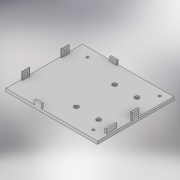
# Autodesk Inventor part: case
Saved by Autodesk Inventor 2019 (Build 230136000, 136)
## iProperties
Created: 2020-05-08
Part Number: case
Material: Generic
Document SubType Name: Modeling
Designer: Mateusz
Density: 1 g/cm^3
Appearance: Default
Author: Mateusz
Autodesk Inventor part; units mm, degrees
ref_plane "YZ Plane" through (0, 0, 0) normal (1, 0, 0) x (0, 1, 0)
ref_plane "XZ Plane" through (0, 0, 0) normal (0, 1, 0) x (-1, 0, 0)
ref_plane "XY Plane" through (0, 0, 0) normal (0, 0, 1) x (1, 0, 0)
sketch "Sketch1" plane through (0, 0, 0) normal (0, 1, 0) x (-1, 0, 0)
  line L0 (0, 0) -> (0, 98.75)
  line L1 (0, 98.75) -> (114.73, 98.75)
  line L2 (114.73, 98.75) -> (114.73, 0)
  line L3 (114.73, 0) -> (0, 0)
  line L4 (0, 98.75) -> (0, 90.47)
  circle A0 centre (11.7, 90.47) radius 1.65
  line L5 (0, 0) -> (0, 6.72)
  circle A1 centre (6.58, 6.72) radius 1.65
  line L6 (114.73, 0) -> (114.73, 9.87)
  circle A2 centre (100.11, 9.87) radius 1.65
  line L7 (-2, 0) -> (-2, 98.75)
  line L8 (-2, 98.75) -> (-2, 100.75)
  line L9 (-2, 100.75) -> (114.73, 100.75)
  line L10 (114.73, 100.75) -> (116.73, 100.75)
  line L11 (116.73, 100.75) -> (116.73, 0)
  line L12 (116.73, 0) -> (116.73, -2)
  line L13 (116.73, -2) -> (-2, -2)
  line L14 (-2, -2) -> (-2, 0)
  dimension "d11" = 2
  dimension "d12" = 2
  dimension "d13" = 2
  dimension "d14" = 2
  constraints: 30 end point, 7 point on line, 6 perpendicular, 3 centre point, 1 horizontal, 1 vertical
  measures "d11" distance of L0.start L7.start
  measures "d12" distance of L7.end L8.end
  measures "d13" distance of L9.end L10.end
  measures "d14" distance of L11.end L12.end
extrude "Extrusion1" add sketch "Sketch1" along normal blind 4 contours L0 L1 L2 L3 | L7 L8 L9 L10 L11 L12 L13 L14
sketch "Sketch9" plane through (0, 4, 0) normal (0, 1, 0) x (1, 0, 0)
  circle A0 centre (-50, -75.0625) radius 1.65
  circle A1 centre (-20, -75.0625) radius 1.65
  circle A2 centre (-50, -23.6875) radius 1.65
  circle A3 centre (-20, -23.6875) radius 1.65
  point P0 (2, 2)
  dimension "d51" = 3.3
  dimension "d52" = 3.3
  dimension "d54" = 3.3
  dimension "d55" = 3.3
  constraints: 4 centre point
  measures "d51" diameter of A0
  measures "d52" diameter of A1
  measures "d54" diameter of A2
  measures "d55" diameter of A3
extrude "Extrusion9" cut sketch "Sketch9" against normal blind 10
sketch "Sketch10" plane through (0, 4, 0) normal (0, 1, 0) x (1, 0, 0)
  circle A0 centre (-50, -75.0625) radius 1.65 projected
  circle A1 centre (-50, -75.0625) radius 3
  circle A2 centre (-50, -23.6875) radius 1.65 projected
  circle A3 centre (-50, -23.6875) radius 3
  circle A4 centre (-20, -23.6875) radius 1.65 projected
  circle A5 centre (-20, -23.6875) radius 3
  circle A6 centre (-20, -75.0625) radius 1.65 projected
  circle A7 centre (-20, -75.0625) radius 3
  point P0 (0, 0)
  dimension "d58" = 6
  dimension "d59" = 6
  dimension "d60" = 6
  dimension "d61" = 6
  constraints: 4 centre point, 4 coincident
  measures "d58" diameter of A1
  measures "d59" diameter of A3
  measures "d60" diameter of A5
  measures "d61" diameter of A7
extrude "Extrusion10" cut sketch "Sketch10" against normal blind 2
sketch "Sketch11" plane through (-116.73, 0, -2) normal (-1, 0, 0) x (0, 0, 1)
  line L0 (0, 0) -> (102.75, 0) projected
  line L1 (102.75, 4) -> (0, 4) projected
  line L2 (102.75, 0) -> (102.75, 4)
  line L3 (102.75, 4) -> (0, 4)
  line L4 (0, 0) -> (0, 4) projected
  line L5 (0, 4) -> (0, 0)
  line L6 (0, 0) -> (102.75, 0)
  point P0 (2, 0)
  constraints: 8 end point, 2 perpendicular, 1 collinear, 1 vertical
extrude "Extrusion11" add sketch "Sketch11" along normal blind 2
sketch "Sketch12" plane through (0, 4, 0) normal (0, 1, 0) x (1, 0, 0)
  line L0 (-118.73, -100.75) -> (-118.73, 2) projected
  line L1 (-118.73, -100.75) -> (-118.73, -80.75)
  line L2 (-118.73, -80.75) -> (-116.73, -80.75)
  line L3 (-116.73, -80.75) -> (-116.73, -70.75)
  line L4 (-116.73, -70.75) -> (-118.73, -70.75)
  line L5 (-118.73, -80.75) -> (-118.73, -70.75)
  line L6 (-118.73, 2) -> (-118.73, -18)
  line L7 (-118.73, -18) -> (-116.73, -18)
  line L8 (-116.73, -18) -> (-116.73, -28)
  line L9 (-116.73, -28) -> (-118.73, -28)
  line L10 (-118.73, -18) -> (-118.73, -28)
  point P0 (0, 0)
  dimension "d66" = 20
  dimension "d67" = 2
  dimension "d68" = 10
  dimension "d69" = 20
  dimension "d70" = 2
  dimension "d71" = 10
  constraints: 20 end point, 6 point on line, 4 perpendicular, 2 collinear
  measures "d66" distance of L0.start L1.end
  measures "d67" distance of L1.end L2.end
  measures "d68" distance of L2.end L3.end
  measures "d69" distance of L0.end L6.end
  measures "d70" distance of L6.end L7.end
  measures "d71" distance of L7.end L8.end
extrude "Extrusion12" add sketch "Sketch12" along normal blind 10
sketch "Sketch13" plane through (-118.73, 0, -2) normal (-1, 0, 0) x (0, 0, 1)
  line L0 (20, 14) -> (30, 14) projected
  line L1 (25, 14) -> (25, 9)
  line L2 (82.75, 14) -> (72.75, 14) projected
  line L3 (77.75, 14) -> (77.75, 9)
  circle A0 centre (25, 9) radius 1.65
  circle A1 centre (77.75, 9) radius 1.65
  point P0 (2, 0)
  dimension "d74" = 5
  dimension "d77" = 3.3
  dimension "d78" = 3.3
  constraints: 4 end point, 2 centre point, 2 coincident, 2 midpoint, 2 vertical
  measures "d74" distance of L1.start L1.end
  measures "d77" diameter of A0
  measures "d78" diameter of A1
sketch "Sketch14" plane through (2, 0, 100.75) normal (1, 0, 0) x (0, 0, -1)
  line L0 (0, 4) -> (102.75, 4) projected
  line L1 (0, 0) -> (0, 4) projected
  line L2 (0, 4) -> (0, 0)
  line L3 (102.75, 0) -> (102.75, 4) projected
  line L4 (0, 0) -> (102.75, 0)
  line L5 (102.75, 0) -> (102.75, 4)
  line L6 (102.75, 4) -> (0, 4)
  point P0 (100.75, 0)
  constraints: 8 end point, 2 collinear, 2 perpendicular
extrude "Extrusion13" add sketch "Sketch14" along normal blind 2
sketch "Sketch15" plane through (0, 4, 0) normal (0, 1, 0) x (1, 0, 0)
  line L0 (4, 2) -> (4, -100.75) projected
  line L1 (2, -49.375) -> (2, -44.375)
  line L2 (2, -44.375) -> (4, -44.375)
  line L3 (2, -49.375) -> (2, -54.375)
  line L4 (2, -54.375) -> (4, -54.375)
  line L5 (4, -44.375) -> (4, -44.7728)
  line L6 (4, -54.375) -> (4, -44.375)
  point P0 (0, 0)
  dimension "d82" = 5
  dimension "d83" = 5
  constraints: 12 end point, 3 point on line, 2 perpendicular, 1 collinear, 1 vertical
  measures "d82" distance of L1.start L1.end
  measures "d83" distance of L1.start L3.end
extrude "Extrusion14" add sketch "Sketch15" along normal blind 10
sketch "Sketch16" plane through (4, 0, 100.75) normal (1, 0, 0) x (0, 0, -1)
  line L0 (56.375, 14) -> (46.375, 14) projected
  line L1 (51.375, 14) -> (51.375, 9)
  circle A0 centre (51.375, 9) radius 1.65
  point P0 (100.75, 0)
  dimension "d86" = 5
  dimension "d87" = 3.3
  constraints: 2 end point, 1 centre point, 1 coincident, 1 midpoint, 1 vertical
  measures "d86" distance of L1.start L1.end
  measures "d87" diameter of A0
extrude "Extrusion15" cut sketch "Sketch16" against normal blind 10
extrude "Extrusion16" cut sketch "Sketch13" against normal blind 10
sketch "Sketch17" plane through (0, 4, 0) normal (0, 1, 0) x (1, 0, 0)
  line L0 (-71.73, 2) -> (-71.015, 2)
  line L1 (-71.015, 2) -> (-71.015, 0)
  line L2 (-71.015, 0) -> (-80.015, 0)
  line L3 (-80.015, 2) -> (-80.015, 0)
  line L4 (-80.015, 2) -> (-71.73, 2)
  line L5 (-118.73, 2) -> (4, 2) projected
  line L6 (-80.015, -100.75) -> (-80.015, -98.75)
  line L7 (-71.73, -98.75) -> (-71.015, -98.75)
  line L8 (-71.015, -98.75) -> (-71.015, -100.75)
  line L9 (-71.015, -100.75) -> (-80.015, -100.75)
  line L10 (-80.015, -98.75) -> (-71.73, -98.75)
  point P0 (0, 0)
  point P1 (-118.73, -100.75)
  dimension "d107" = 0.715
  dimension "d109" = 0.715
  constraints: 20 end point, 2 perpendicular, 1 collinear, 1 horizontal
  measures "d107" distance of L0.start L0.end
  measures "d109" distance of L7.start L7.end
extrude "Extrusion17" add sketch "Sketch17" along normal blind 6
sketch "Sketch18" plane through (0, 4, 0) normal (0, 1, 0) x (1, 0, 0)
  line L0 (4, -54.375) -> (4, -100.75) projected
  line L1 (4, -100.75) -> (4, -86.75)
  line L2 (4, -86.75) -> (4, -72.75)
  line L3 (4, -72.75) -> (0, -72.75)
  line L4 (0, -72.75) -> (0, -86.75)
  line L5 (0, -86.75) -> (2, -86.75)
  line L6 (2, -86.75) -> (2, -72.75)
  point P0 (0, 0)
  dimension "d100" = 14
  dimension "d101" = 14
  dimension "d102" = 4
  dimension "d103" = 2
  constraints: 12 end point, 3 perpendicular, 2 point on line, 1 midpoint
  measures "d100" distance of L0.end L1.end
  measures "d101" distance of L1.end L2.end
  measures "d102" distance of L2.end L3.end
  measures "d103" distance of L4.end L5.end
extrude "Extrusion18" add sketch "Sketch18" along normal blind 6
fillet "Fillet1" radius 1 9 edges at (4, 14, 49.375) (4, 9, 44.375) (4, 9, 54.375) (4, 4, 21.1875) (-118.73, 9, 80.75) (-118.73, 14, 75.75) (-118.73, 9, 70.75) (-118.73, 14, 23) (-118.73, 9, 18)
fillet "Fillet2" radius 1 2 edges at (-118.4371, 13.7071, 28) (-118.73, 8.5, 28)
body "Solid1"
